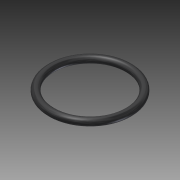
# Autodesk Inventor part: Rebuild Shooter NCDME075-0600 Piston Seal
Saved by Autodesk Inventor 2014 SP1 (Build 180222100, 222)
## iProperties
Created: 2013-12-20
Part Number: Rebuild Shooter NCDME075-0600 Piston Seal
Material: Rubber
Document SubType Name: Modeling
Designer: Moses
Density: 0.93 g/cm^3
Appearance: Rubber - Black - Version 1.1
Mass: 0.100985 g
Surface Area: 2.73602 cm^2
Volume: 0.108586 cm^3
Author: Moses
Autodesk Inventor part; units mm, degrees
ref_plane "YZ Plane" through (0, 0, 0) normal (1, 0, 0) x (0, 1, 0)
ref_plane "XZ Plane" through (0, 0, 0) normal (0, 1, 0) x (-1, 0, 0)
ref_plane "XY Plane" through (0, 0, 0) normal (0, 0, 1) x (1, 0, 0)
sketch "Sketch1" plane through (0, 0, 0) normal (0, 0, 1) x (1, 0, 0)
  line L0 (0, 0) -> (8.7312, 0) construction
  circle A0 centre (8.7312, 0) radius 0.7937
  line L1 (0, 0) -> (0, -2.54)
  dimension "d0" = 8.7312
  dimension "d1" = 1.5875
  dimension "d2" = 2.54
  constraints: 4 end point, 1 centre point, 1 coincident, 1 horizontal, 1 vertical
  measures "d0" distance of L0.start L0.end
  measures "d1" diameter of A0
  measures "d2" distance of L0.start L1.end
revolve "Revolution1" add sketch "Sketch1" angle 360 about axis through (0, 0, 0) along (0, -1, 0)
body "Solid1"
